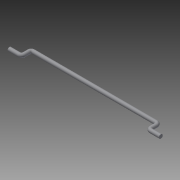
# Autodesk Inventor part: rotobot pushrod
Saved by Autodesk Inventor 2015 SP2 (Build 190223200, 223)
## iProperties
Created: 2015-05-25
Part Number: rotobot pushrod
Material: Generic
Document SubType Name: Modeling
Designer: caleb
Density: 1 g/cm^3
Appearance: Default
Author: caleb
Autodesk Inventor part; units mm, degrees
ref_plane "XZ Plane" through (0, 0, 0) normal (0, 1, 0) x (-1, 0, 0)
ref_plane "XY Plane" through (0, 0, 0) normal (0, 0, 1) x (1, 0, 0)
sketch "Sketch1" plane through (0, 0, 0) normal (0, 0, 1) x (1, 0, 0)
  line L0 (0, 0) -> (12.7, 0)
  arc A0 (13.2, -0.5) -> (12.7, 0) centre (12.7, -0.5) ccw
  line L1 (13.2, -0.5) -> (13.2, -1.5)
  arc A1 (13.2, -1.5) -> (13.7, -2) centre (13.7, -1.5) ccw
  line L2 (13.7, -2) -> (15.7, -2)
  dimension "d0" = 0.5
  dimension "d1" = 2
  dimension "d2" = 90
  dimension "d3" = 12.7
  dimension "d5" = 2
  constraints: 6 end point, 4 point on circle, 4 tangent, 2 centre point, 2 horizontal, 1 equal radius
  measures "d0" radius of A1
  measures "d1" distance between parallel lines of L0 L2
  measures "d2" angle of L1 L0
  measures "d3" distance of L0.start L0.end
  measures "d5" distance of L2.start L2.end
ref_plane "Work Plane2" through (15.7, -2, 0) normal (1, 0, 0) x (0, 1, 0)
sketch "Sketch3" plane through (15.7, -2, 0) normal (1, 0, 0) x (0, 1, 0)
  circle A0 centre (0, 0) radius 0.4
  point P0 (2, 0)
  dimension "d6" = 0.8
  constraints: 1 centre point, 1 coincident
  measures "d6" diameter of A0
sweep "Sweep1" add profiles "Sketch3" path "Sketch1"
mirror "Mirror1" about plane through (0, 0, 0) normal (-1, 0, 0) of "Sweep1"
body "Solid1"
